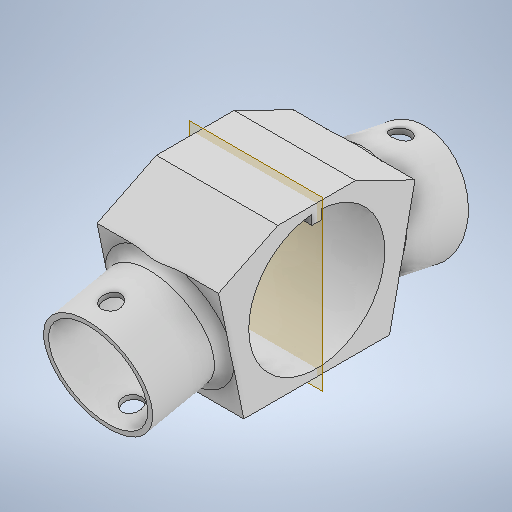
# Autodesk Inventor part: bielle côté 3
Saved by Autodesk Inventor 2026.2 (Build 302298010, 298A)
## iProperties
Created: 2026-03-16
Part Number: bielle côté 3
Material: Générique
Document SubType Name: Modeling
Designer: genon
Density: 1 g/cm^3
Appearance: Par défaut
Author: genon
Autodesk Inventor part; units mm, degrees
ref_plane "YZ Plane" through (0, 0, 0) normal (1, 0, 0) x (0, 1, 0)
ref_plane "XZ Plane" through (0, 0, 0) normal (0, 1, 0) x (-1, 0, 0)
sketch "Esquisse1" plane through (0, 0, 0) normal (1, 0, 0) x (0, 1, 0)
  line L0 (0, 0) -> (0, -15)
  line L1 (0, 0) -> (0, 15)
  line L2 (0, 0) -> (15.5, 0)
  circle A0 centre (15.5, 0) radius 14
  line L3 (0, 0) -> (31, 0)
  line L4 (31, 0) -> (31, 8)
  line L5 (31, 0) -> (31, -8)
  line L6 (29.5, 0) -> (27.5, 0)
  line L7 (27.5, 0) -> (27.5, -1)
  line L8 (27.5, -1) -> (29.4642, -1)
  line L9 (27.5, 0) -> (27.5, 1)
  line L10 (27.5, 1) -> (29.4642, 1)
  line L11 (31, 8) -> (25, 20.2269)
  line L12 (0, 15) -> (25, 20.2269)
  line L13 (31, -8) -> (25, -20.2269)
  line L14 (0, -15) -> (25, -20.2269)
  dimension "d0" = 15
  dimension "d1" = 15
  dimension "d3" = 15.5
  dimension "d4" = 28
  dimension "d5" = 31
  dimension "d6" = 8
  dimension "d8" = 1
  dimension "d9" = 1
  dimension "d17" = 25
  dimension "d18" = 5.2269
  constraints: 30 end point, 4 perpendicular, 3 point on circle, 3 point on line, 3 vertical, 2 symmetric about line, 1 centre point, 1 coincident, 1 horizontal
  measures "d0" distance of L0.start L0.end
  measures "d1" distance of L0.start L1.end
  measures "d3" distance of L0.start L2.end
  measures "d4" diameter of A0
  measures "d5" distance of L0.start L3.end
  measures "d6" distance of L3.end L4.end
  measures "d8" distance of L6.end L7.end
  measures "d9" distance of L6.end L9.end
  measures "d17" horizontal distance of L1.end L11.end
  measures "d18" vertical distance of L11.end L1.end
extrude "Extrusion1" add sketch "Esquisse1" along normal blind 25 contours L2 A0 L3 L5 L13 L14 L0 | L1 L12 L11 L4 L3 A0 L2 | A0 L3 L9 L10 | L8 L7 L3 A0
sketch "Esquisse5" plane through (0, 0, 15) normal (0, -0.2046524, 0.9788347) x (1, 0, 0)
  line L0 (0, 0) -> (25, 0) projected
  line L1 (0, 25.5406) -> (25, 25.5406) projected
  circle A0 centre (12.5, 13.7247) radius 10
  circle A1 centre (12.5, 13.7247) radius 11
  line L2 (12.5, 13.7247) -> (12.5, 0)
  point P0 (0, -3.0698)
  dimension "d21" = 20
  dimension "d22" = 22
  dimension "d27" = 13.7247
  constraints: 2 centre point, 2 end point, 1 coincident, 1 midpoint
  measures "d21" diameter of A0
  measures "d22" diameter of A1
  measures "d27" distance of L2.start L2.end
extrude "Extrusion3" add sketch "Esquisse5" along normal blind 15
fillet "Congé1" radius 2 1 edges at (1.5, 13.4342, 17.8088)
sketch "Esquisse7" plane through (25, 25, -20.2269) normal (0, -0.2046524, -0.9788347) x (-1, 0, 0)
  line L0 (25, -25.5406) -> (0, -25.5406) projected
  line L1 (12.5, -25.5406) -> (12.5, -11.8159)
  circle A0 centre (12.5, -11.8159) radius 10
  circle A1 centre (12.5, -11.8159) radius 11
  point P0 (25, -28.6104)
  dimension "d28" = 13.7247
  dimension "d29" = 20
  dimension "d30" = 22
  constraints: 2 centre point, 2 coincident, 2 end point, 1 midpoint, 1 vertical
  measures "d28" distance of L1.start L1.end
  measures "d29" diameter of A0
  measures "d30" diameter of A1
extrude "Extrusion4" add sketch "Esquisse7" along normal blind 15
fillet "Congé2" radius 2 1 edges at (23.5, 13.4342, -17.8088)
ref_plane "Plan de construction5" through (0, 0, 0) normal (0, -0.9788347, -0.2046524) x (1, 0, 0)
sketch "Esquisse8" plane through (0, 0, 0) normal (0, -0.9788347, -0.2046524) x (1, 0, 0)
  line L0 (1.5, 16.6825) -> (1.5, 29.6825) projected
  line L1 (1.5, 29.6825) -> (12.5, 29.6825)
  line L2 (23.5, 16.6825) -> (23.5, 29.6825) projected
  line L3 (12.5, 29.6825) -> (12.5, 24.6825)
  point P0 (0, 0)
  dimension "d35" = 11
  dimension "d36" = 5
  constraints: 4 end point, 1 coincident, 1 parallel, 1 perpendicular, 1 point on line
  measures "d35" distance of L1.start L1.end
  measures "d36" distance of L1.end L3.end
hole "Perçage1" at (12.5, -5.0513, 24.1601) direction (0, 0.9788347, 0.2046524) diameter 4 end through all
ref_plane "Plan de construction6" through (0, 0, 0) normal (0, 0.9788347, -0.2046524) x (1, 0, 0)
sketch "Esquisse9" plane through (0, 0, 0) normal (0, 0.9788347, -0.2046524) x (1, 0, 0)
  line L0 (23.5, 29.6825) -> (1.5, 29.6825) projected
  line L1 (23.5, 29.6825) -> (12.5, 29.6825)
  line L2 (12.5, 29.6825) -> (12.5, 24.6825)
  point P0 (0, 0)
  dimension "d45" = 11
  dimension "d46" = 5
  constraints: 4 end point, 1 coincident, 1 midpoint, 1 perpendicular
  measures "d45" distance of L0.start L1.end
  measures "d46" distance of L1.end L2.end
hole "Perçage2" at (12.5, -5.0513, -24.1601) direction (0, 0.9788347, -0.2046524) diameter 4 end through all
